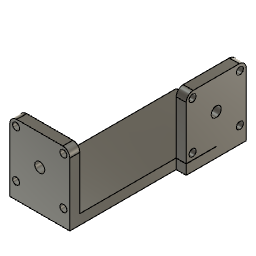
braco-finalizado (Autodesk Fusion 360 archive; units mm, degrees)
design "EngrenagemBracoFinal v2"
Autodesk Fusion 360 part; units mm, degrees
sketch "Sketch1" plane through (0, 0, 0) normal (0, 1, 0) x (1, 0, 0)
  line L0 (23.622, -23.622) -> (-23.622, -23.622)
  line L1 (-23.622, -23.622) -> (-23.622, 23.622)
  line L2 (-23.622, 23.622) -> (23.622, 23.622)
  line L3 (23.622, 23.622) -> (23.622, -23.622)
  line L4 (23.622, -23.622) -> (-23.622, 23.622) construction
  line L5 (-23.622, -23.622) -> (23.622, 23.622) construction
  circle A0 centre (-23.622, -23.622) radius 3.5
  circle A1 centre (23.622, -23.622) radius 3.5
  circle A2 centre (-23.622, 23.622) radius 3.5
  circle A3 centre (23.622, 23.622) radius 3.5
  circle A4 centre (0, 0) radius 5
  line L6 (0, 0) -> (30, 0)
  line L7 (30, 0) -> (30, -23)
  line L8 (23, -30) -> (0, -30)
  line L9 (0, -30) -> (0, 0)
  line L10 (0, 0) -> (-30, 0)
  line L11 (-30, 0) -> (-30, -23)
  line L12 (-23, -30) -> (0, -30)
  line L13 (0, -30) -> (0, 0)
  line L14 (0, 0) -> (-30, 0)
  line L15 (-30, 0) -> (-30, 30)
  line L16 (-30, 30) -> (0, 30)
  line L17 (0, 30) -> (0, 0)
  line L18 (0, 0) -> (30, 0)
  line L19 (30, 0) -> (30, 30)
  line L20 (30, 30) -> (0, 30)
  line L21 (0, 30) -> (0, 0)
  line L22 (-30, 30) -> (-30, 40)
  line L23 (-30, 40) -> (30, 40)
  line L24 (30, 40) -> (30, 30)
  line L25 (30, -30) -> (40, -30)
  line L26 (40, -30) -> (40, 40)
  arc A5 (-30, -23) -> (-23, -30) centre (-23, -23) ccw
  arc A6 (23, -30) -> (30, -23) centre (23, -23) ccw
  line L27 (30, -23) -> (30, -30)
  line L28 (40, 40) -> (30, 40)
  dimension "d1" = 47.244
  dimension "d2" = 47.244
  dimension "d3" = 7
  dimension "d4" = 7
  dimension "d5" = 7
  dimension "d6" = 7
  dimension "d7" = 10
  dimension "d8" = 10
  dimension "d9" = 7
  constraint horizontal L0
  constraint perpendicular L0 L1
  constraint parallel L0 L2
  constraint parallel L1 L3
  constraint coincident L4 A4.centre
  constraint coincident L5 A4.centre
  constraint coincident A4.centre L6.start
  constraint coincident L0.end L1.start
  constraint coincident L0.start L3.end
  constraint coincident L1.end L2.start
  constraint coincident L2.end L3.start
  constraint horizontal L6
  constraint vertical L7
  constraint horizontal L8
  constraint vertical L9
  constraint horizontal L10
  constraint vertical L11
  constraint horizontal L12
  constraint vertical L13
  constraint horizontal L14
  constraint vertical L15
  constraint horizontal L16
  constraint vertical L17
  constraint horizontal L18
  constraint vertical L19
  constraint horizontal L20
  constraint vertical L21
  constraint perpendicular L16 L22
  constraint perpendicular L15 L23
  constraint perpendicular L20 L24
  constraint perpendicular L7 L25
  constraint perpendicular L25 L26
  constraint tangent L11 A5
  constraint tangent L12 A5
  constraint coincident L25.start L8
  constraint coincident L25.start L7
  constraint tangent L8 A6
  constraint tangent L7 A6
  constraint equal A5 A6
  constraint perpendicular L24 L28
  measures "d1" distance of L1.end L2.end
  measures "d2" distance of L0 L2
  measures "d3" diameter of A0
  measures "d4" diameter of A1
  measures "d5" diameter of A2
  measures "d6" diameter of A3
  measures "d7" diameter of A4
  measures "d8" distance of L25.start L25.end
  measures "d9" radius of A5
extrude "Extrude2" add sketch "Sketch1" along normal blind 180 contours L0 L1 A0 A4 L9 L10 L13 L14 | L0 L1 A0 L9 L10 L11 L12 L13 L14 A5 | L0 L3 A1 A4 L6 L9 L13 L18 | L0 L3 A1 L6 L7 L8 L9 L13 L18 A6 | L1 L2 A2 L10 L14 L15 L16 L17 L21 | L1 L2 A2 A4 L10 L14 L17 L21 | L2 L3 A3 A4 L6 L17 L18 L21 | L2 L3 A3 L6 L17 L18 L19 L20 L21 | L7 L19 L24 L25 L26 L27 L28 | L16 L20 L22 L23 L24
sketch "Sketch2" plane through (0, 0, 0) normal (0, 1, 0) x (1, 0, 0)
  line L0 (40, 40) -> (30, 40)
  dimension "d12" = 10
  constraint horizontal L0
  measures "d12" distance of L0.start L0.end
sketch "Sketch3" plane through (0, 180, 0) normal (0, 1, 0) x (-1, 0, 0)
  circle A0 centre (23.622, 23.622) radius 3.5
  circle A1 centre (23.622, -23.622) radius 3.5
  circle A2 centre (0, 0) radius 5
  circle A3 centre (-23.622, -23.622) radius 3.5
  circle A4 centre (-23.622, 23.622) radius 3.5
  arc A5 (-23, 30) -> (-30, 23) centre (-23, 23) ccw
  line L0 (-30, 23) -> (-30, 30)
  line L1 (-30, 30) -> (-40, 30)
  line L2 (-40, 30) -> (-40, -40)
  line L3 (-40, -40) -> (30, -40)
  line L4 (30, -40) -> (30, 23)
  arc A6 (30, 23) -> (23, 30) centre (23, 23) ccw
  line L5 (23, 30) -> (-23, 30)
  line L6 (23.622, 23.622) -> (-23.622, 23.622)
  line L7 (-23.622, 23.622) -> (-23.622, -23.622)
  line L8 (-23.622, -23.622) -> (23.622, -23.622)
  line L9 (23.622, -23.622) -> (23.622, 23.622)
  line L10 (23.622, 23.622) -> (-23.622, -23.622) construction
  line L11 (-23.622, 23.622) -> (23.622, -23.622) construction
  circle A7 centre (-23.622, 23.622) radius 3.5
  circle A8 centre (23.622, 23.622) radius 3.5
  circle A9 centre (-23.622, -23.622) radius 3.5
  circle A10 centre (23.622, -23.622) radius 3.5
  circle A11 centre (0, 0) radius 5
  line L12 (23, 30) -> (-23, 30)
  line L13 (-30, 30) -> (-30, -30)
  line L14 (-30, -30) -> (30, -30)
  line L15 (30, -30) -> (30, 23)
  line L16 (30, 30) -> (-30, -30) construction
  line L17 (-30, 30) -> (30, -30) construction
  arc A12 (30, 23) -> (23, 30) centre (23, 23) ccw
  line L18 (-30, 30) -> (-40, 30)
  line L19 (-40, -40) -> (30, -40)
  line L20 (-30, 23) -> (-30, 0)
  arc A13 (-23, 30) -> (-30, 23) centre (-23, 23) ccw
  dimension "d15" = 7
  dimension "d16" = 7
  dimension "d17" = 7
  dimension "d18" = 7
  dimension "d19" = 10
  dimension "d20" = 60
  dimension "d21" = 7
  dimension "d22" = 7
  constraint horizontal L6
  constraint perpendicular L6 L7
  constraint parallel L6 L8
  constraint parallel L7 L9
  constraint coincident L10 A2.centre
  constraint coincident L11 A2.centre
  constraint coincident A0.centre L6.start
  constraint coincident A2.centre A11.centre
  constraint coincident A4.centre L6.end
  constraint coincident A3.centre L7.end
  constraint coincident A1.centre L8.end
  constraint horizontal L12
  constraint perpendicular L12 L13
  constraint parallel L12 L14
  constraint parallel L13 L15
  constraint coincident L16 A2.centre
  constraint coincident L17 A2.centre
  constraint coincident L16.start L12
  constraint coincident L16.start L15
  constraint tangent L12 A12
  constraint tangent L15 A12
  constraint coincident L1.end L2.start
  constraint perpendicular L2 L18
  constraint coincident L2.end L3.start
  constraint coincident L3.end L4.start
  constraint midpoint L13 L20.end
  constraint coincident L0.end L12
  constraint coincident L0.end L20
  constraint tangent L12 A13
  constraint tangent L20 A13
  measures "d15" diameter of A7
  measures "d16" diameter of A8
  measures "d17" diameter of A9
  measures "d18" diameter of A10
  measures "d19" diameter of A11
  measures "d20" distance of L13.end L14.end
  measures "d21" radius of A12
  measures "d22" radius of A13
extrude "Extrude3" cut sketch "Sketch3" against normal blind 170 contours A0 A1 A3 A4 L6 L7 L8 L9 A7 A8 A9 A10 | A5 L4 A6 L5 L12 L13 L14 L15 A12 L20 A13
move_body "Move1" bodies 1 to x (1, 0, 0) y (0, 1, 0) z (0, 0, 1) at (92.495, 0, 81.1548)
sketch "Sketch4" plane through (0, 0, 0) normal (1, 0, 0) x (0, 1, 0)
sketch "Sketch5" plane through (0, 180, 0) normal (0, 1, 0) x (-1, 0, 0)
  line L0 (-62.495, 51.1548) -> (-122.495, 51.1548)
  line L1 (-122.495, 51.1548) -> (-122.495, 111.1548)
  line L2 (-122.495, 111.1548) -> (-132.495, 111.1548)
  line L3 (-132.495, 111.1548) -> (-132.495, 41.1548)
  line L4 (-132.495, 41.1548) -> (-62.495, 41.1548)
  line L5 (-62.495, 41.1548) -> (-62.495, 51.1548)
  line L6 (-122.495, 111.1548) -> (-122.495, 44)
  line L7 (-122.495, 44) -> (-122.495, 41.1548)
  line L8 (-132.495, 41.1548) -> (-132.495, 65)
  line L9 (-132.495, 65) -> (-132.495, 111.1548)
  constraint coincident L1.end L2.start
  constraint perpendicular L4 L6
  constraint coincident L4 L7.end
  constraint perpendicular L4 L7
  constraint coincident L3.end L4.start
  constraint coincident L3 L8.end
  constraint perpendicular L4 L8
  constraint coincident L2.end L3.start
extrude "Extrude4" cut sketch "Sketch5" against normal blind 200 contours L1 L2 L3 L4 L6 L7 L8 L9
sketch "Sketch6" plane through (122.495, 0, 0) normal (1, 0, 0) x (0, 1, 0)
  line L0 (0, 104.1548) -> (0, 41.1548)
  line L1 (0, 41.1548) -> (180, 41.1548)
  line L2 (180, 41.1548) -> (180, 51.1548)
  line L3 (180, 51.1548) -> (10, 51.1548)
  line L4 (10, 51.1548) -> (10, 104.1548)
  line L5 (10, 104.1548) -> (0, 104.1548)
  line L6 (180, 41.1548) -> (180, 120)
  line L7 (180, 120) -> (166.2247, 120)
  line L8 (166.2247, 104.1273) -> (166.2247, 41.1548)
  line L9 (106.4269, 111.1273) -> (106.2247, 111.1273)
  line L10 (113.2247, 111.1273) -> (159.2247, 111.1273)
  line L11 (166.2247, 111.1273) -> (190, 111.1273)
  line L12 (100, 81.1548) -> (200, 81.1548)
  line L13 (106.2247, 104.1273) -> (106.2247, 33.1392)
  line L14 (136.2247, 140) -> (136.2247, 30)
  line L15 (159.8632, 104.7933) -> (112.5862, 104.7933)
  line L16 (112.5862, 104.7933) -> (112.5862, 57.5163)
  line L17 (112.5862, 57.5163) -> (159.8632, 57.5163)
  line L18 (159.8632, 57.5163) -> (159.8632, 104.7933)
  line L19 (159.8632, 104.7933) -> (112.5862, 57.5163) construction
  line L20 (112.5862, 104.7933) -> (159.8632, 57.5163) construction
  circle A0 centre (112.5862, 104.7933) radius 3.5
  circle A1 centre (159.8632, 104.7933) radius 3.5
  circle A2 centre (159.8632, 57.5163) radius 3.5
  circle A3 centre (112.5862, 57.5163) radius 3.5
  circle A4 centre (136.2247, 81.1548) radius 5
  arc A5 (113.2247, 111.1273) -> (106.2247, 104.1273) centre (113.2247, 104.1273) ccw
  arc A6 (166.2247, 104.1273) -> (159.2247, 111.1273) centre (159.2247, 104.1273) ccw
  line L21 (166.2247, 120) -> (166.2247, 24.7933)
  line L22 (166.2247, 24.7933) -> (190, 24.7933)
  line L23 (190, 24.7933) -> (190, 130)
  line L24 (190, 130) -> (166.2247, 130)
  line L25 (166.2247, 130) -> (166.2247, 90)
  point P0 (136.2247, 81.1548)
  dimension "d27" = 30
  dimension "d28" = 29.9725
  dimension "d29" = 60
  dimension "d30" = 30
  dimension "d31" = 47.277
  dimension "d32" = 47.277
  dimension "d33" = 13.7753
  dimension "d34" = 7
  dimension "d35" = 7
  dimension "d36" = 7
  dimension "d37" = 7
  dimension "d38" = 10
  dimension "d39" = 7
  dimension "d40" = 7
  constraint coincident L1.end L2.start
  constraint perpendicular L3 L6
  constraint perpendicular L2 L7
  constraint coincident L1 L8.end
  constraint perpendicular L1 L8
  constraint horizontal L9
  constraint coincident L8 L11.start
  constraint perpendicular L8 L10
  constraint perpendicular L6 L11
  constraint perpendicular L6 L12
  constraint perpendicular L1 L13
  constraint perpendicular L1 L14
  constraint horizontal L15
  constraint perpendicular L15 L16
  constraint parallel L15 L17
  constraint parallel L16 L18
  constraint coincident L19 P0
  constraint coincident L20 P0
  constraint coincident L12 P0
  constraint coincident L14 P0
  constraint coincident L15.end L16.start
  constraint coincident L15.start L18.end
  constraint coincident L17.end L18.start
  constraint coincident L16.end L17.start
  constraint coincident P0 A4.centre
  constraint coincident L9.end L13
  constraint coincident L9.end L10
  constraint tangent L13 A5
  constraint tangent L10 A5
  constraint coincident L11.start L10
  constraint coincident L7.end L8
  constraint tangent L10 A6
  constraint tangent L8 A6
  constraint perpendicular L1 L21
  constraint perpendicular L21 L22
  constraint perpendicular L22 L23
  constraint perpendicular L21 L24
  constraint coincident L8 L25.end
  constraint perpendicular L24 L25
  measures "d27" distance of L3 L12
  measures "d28" distance of L10 L12
  measures "d29" distance of L8 L13
  measures "d30" distance of L13 L14
  measures "d31" distance of L16.end L17.end
  measures "d32" distance of L15 L17
  measures "d33" distance of L6 L7.end
  measures "d34" diameter of A0
  measures "d35" diameter of A1
  measures "d36" diameter of A2
  measures "d37" diameter of A3
  measures "d38" diameter of A4
  measures "d39" radius of A5
  measures "d40" radius of A6
extrude "Extrude5" cut sketch "Sketch6" against normal blind 110 contours L1 L2 L3 L6 L8 L21 | L1 L2 L6 L12 L21 L22 L23 | L3 L6 L8 L12 L21 | L6 L8 L11 L12 L21 L25 | L6 L11 L12 L23 | L6 L7 L11 L21 L25 | L6 L7 L11 L23 L24 L25
sketch "Sketch7" plane through (122.495, 0, 0) normal (1, 0, 0) x (0, 1, 0)
  line L0 (106.2157, 41.1633) -> (124, 41.1633)
  line L1 (124, 41.1633) -> (166, 41.1633)
  line L2 (166, 41.1633) -> (166, 51)
  line L3 (166, 51) -> (106, 51)
  line L4 (106.2157, 41.1633) -> (106.2157, 51.2468)
  line L5 (106.2157, 51.2468) -> (106.2157, 51.1499)
  line L6 (106.2157, 51.1499) -> (108, 51.1499)
  line L7 (108, 51.1499) -> (166.2252, 51.1545)
  dimension "d43" = 17.7843
  constraint horizontal L0
  constraint parallel L0 L1
  constraint perpendicular L0 L2
  constraint perpendicular L2 L3
  constraint perpendicular L3 L4
  constraint coincident L4 L5.end
  constraint perpendicular L5 L6
  measures "d43" distance of L0.start L0.end
extrude "Extrude6" add sketch "Sketch7" sketch "Sketch6" along normal blind 10 of sketch 2 contours L1 L3 L8 L14 L21 | L3 L12 L13 L14 L16 L17 A3 | L3 L8 L12 L14 L17 L18 A2 L21 | L10 L12 L13 L14 L15 L16 A0 A5 | L12 L14 L16 L17 A3 A4 | L12 L14 L17 L18 A2 A4 | L12 L14 L15 L16 A0 A4 | L8 L10 L12 L14 L15 L18 A1 A6 L21 L25 | L12 L14 L15 L18 A1 A4
move_body "Move2" bodies 1 to x (1, 0, 0) y (0, 1, 0) z (0, 0, 1) at (103.4955, 0, 111.5009)
